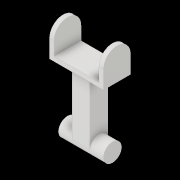
# Autodesk Inventor part: L2_0.1
Saved by Autodesk Inventor 2019 (Build 230136000, 136)
## iProperties
Created: 2021-08-06
Part Number: L2_0.1
Material: ABS 플라스틱
Document SubType Name: Modeling
Designer: YoonJunHeon
Density: 1.06 g/cm^3
Appearance: 매끄러움 - 흰색
Mass: 61056.7 g
Surface Area: 16212.4 cm^2
Volume: 57600.7 cm^3
Author: YoonJunHeon
Autodesk Inventor part; units mm, degrees
ref_plane "YZ Plane" through (0, 0, 0) normal (1, 0, 0) x (0, 1, 0)
ref_plane "XZ Plane" through (0, 0, 0) normal (0, 1, 0) x (-1, 0, 0)
ref_plane "XY Plane" through (0, 0, 0) normal (0, 0, 1) x (1, 0, 0)
sketch "스케치7" plane through (0, 0, 0) normal (1, 0, 0) x (0, 1, 0)
  circle A0 centre (0, 0) radius 10
  dimension "d29" = 20
  constraints: 1 centre point, 1 coincident
  measures "d29" diameter of A0
extrude "돌출7" add sketch "스케치7" along normal mid plane 50
sketch "스케치8" plane through (0, 0, 0) normal (0, 1, 0) x (-1, 0, 0)
  line L0 (25, 10) -> (-25, 10) projected
  line L1 (25, -10) -> (-25, -10) projected
  line L2 (10, 10) -> (-10, 10)
  line L3 (-10, 10) -> (-10, -10)
  line L4 (-10, -10) -> (10, -10)
  line L5 (10, -10) -> (10, 10)
  line L6 (25, -10) -> (25, 10) projected
  point P0 (0, 0)
  dimension "d32" = 20
  dimension "d33" = 15
  constraints: 8 end point, 2 parallel, 2 point on line, 1 horizontal, 1 perpendicular
  measures "d32" distance of L4.end L3.end
  measures "d33" distance between parallel lines of L5 L6
extrude "돌출8" add sketch "스케치8" along normal blind 70 contours L5 L1 L3 L0
sketch "스케치9" plane through (0, 70, 0) normal (0, 1, 0) x (1, 0, 0)
  line L0 (-30, -15) -> (30, -15)
  line L1 (30, -15) -> (30, 15)
  line L2 (30, 15) -> (-30, 15)
  line L3 (-30, 15) -> (-30, -15)
  line L4 (-30, -15) -> (30, 15) construction
  line L5 (30, -15) -> (-30, 15) construction
  point P0 (0, 0)
  dimension "d36" = 60
  dimension "d37" = 30
  constraints: 12 end point, 2 midpoint, 2 parallel, 1 horizontal, 1 perpendicular
  measures "d36" distance of L2.end L1.end
  measures "d37" distance of L1.end L0.end
extrude "돌출9" add sketch "스케치9" along normal blind 5
sketch "스케치10" plane through (-30, 70, -15) normal (-1, 0, 0) x (0, 0, 1)
  line L0 (0, 5) -> (30, 5)
  line L1 (30, 5) -> (30, 20)
  line L2 (30, 20) -> (0, 20)
  line L3 (0, 20) -> (0, 5)
  arc A0 (30, 20) -> (0, 20) centre (15, 20) ccw
  point P0 (15, -70)
  dimension "d40" = 30
  dimension "d41" = 15
  constraints: 8 end point, 2 parallel, 2 point on circle, 1 centre point, 1 horizontal, 1 midpoint, 1 perpendicular
  measures "d40" distance of L2.end L1.end
  measures "d41" distance of L1.end L0.end
extrude "돌출10" add sketch "스케치10" against normal blind 5
mirror "미러3" about plane through (0, 0, 0) normal (1, 0, 0) of "돌출10"
